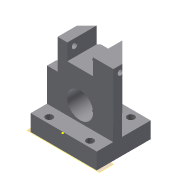
# Autodesk Inventor part: 03_Support_Xslide
Saved by Autodesk Inventor 2019.4 (Build 234330000, 330)
## iProperties
Created: 2021-02-01
Part Number: 03_Support_Xslide
Material: Generic
Document SubType Name: Modeling
Designer: diederichbenedict
Density: 1 g/cm^3
Appearance: Default
Author: diederichbenedict
Autodesk Inventor part; units mm, degrees
ref_plane "YZ Plane" through (0, 0, 0) normal (1, 0, 0) x (0, 1, 0)
ref_plane "XZ Plane" through (0, 0, 0) normal (0, 1, 0) x (-1, 0, 0)
ref_plane "XY Plane" through (0, 0, 0) normal (0, 0, 1) x (1, 0, 0)
ref_plane "Work Plane5" through (16.1538, -3.6432, -7.1) normal (0.0029789, 0.9999956, 0) x (0, 0, 1)
sketch "Sketch5" plane through (16.1538, -3.6432, -7.1) normal (0.0029789, 0.9999956, 0) x (0, 0, 1)
  circle A0 centre (-16.4, -26.2) radius 1.75 projected
  circle A1 centre (-16.4, -6.2) radius 1.75 projected
  line L0 (0, -32.4) -> (6.5, -32.4) projected
  line L1 (6.5, 0) -> (6.5, -32.4) projected
  line L2 (0, 0) -> (6.5, 0) projected
  line L3 (0, 0) -> (0, -32.4) projected
  circle A2 centre (3.6, -6.2) radius 1.75 projected
  circle A3 centre (3.6, -26.2) radius 1.75 projected
  line L4 (-19.9, 0) -> (-19.9, -32.4) projected
  line L5 (6.5, -32.4) -> (-19.9, -32.4)
  line L6 (-19.9, -32.4) -> (-19.9, 0)
  line L7 (-19.9, 0) -> (6.5, 0)
  line L8 (6.5, 0) -> (6.5, -32.4)
  point P0 (7.1, -16.1645)
  constraints: 8 end point, 2 parallel, 1 horizontal, 1 perpendicular
extrude "Extrusion4" add sketch "Sketch5" along normal blind 8
sketch "Sketch7" plane through (16.1776, 4.3568, -7.1) normal (0.0029789, 0.9999956, 0) x (0.9999956, -0.0029789, 0)
  point P0 (-16.1645, -7.1)
sketch "Sketch8" plane through (16.1776, 4.3568, -7.1) normal (0.0029789, 0.9999956, 0) x (0.9999956, -0.0029789, 0)
  circle A0 centre (-26.2, -3.6) radius 1.75 projected
  circle A1 centre (-6.2, -3.6) radius 1.75 projected
  circle A2 centre (-6.2, 16.4) radius 1.75 projected
  circle A3 centre (-26.2, 16.4) radius 1.75 projected
  line L0 (-32.4, -6.5) -> (0, -6.5) projected
  line L1 (0, -6.5) -> (0, 19.9) projected
  line L2 (0, 19.9) -> (-32.4, 19.9) projected
  line L3 (-32.4, 19.9) -> (-32.4, -6.5) projected
  circle A4 centre (-16.2177, 39.3896) radius 1.75 projected
  line L4 (-22.2006, -0.6104) -> (-22.0458, -0.6104) projected
  line L5 (-22.2, -0.6104) -> (-22.2, -0.6104) projected
  line L6 (-22.2, -0.6104) -> (-21.7015, -0.6104) projected
  line L7 (-21.7015, -0.6104) -> (-14.6224, -0.6104) projected
  line L8 (-14.6224, -0.6104) -> (-13.8248, -0.6104) projected
  line L9 (-13.8248, -0.6104) -> (-10.7339, -0.6104) projected
  line L10 (-10.7339, -0.6104) -> (-10.2354, -0.6104) projected
  line L11 (-10.2354, -0.6104) -> (-10.2354, -0.6104) projected
  line L12 (-10.3901, -0.6104) -> (-10.2354, -0.6104) projected
  line L13 (-10.966, -0.6104) -> (-10.3901, -0.6104) projected
  line L14 (-11.1588, -0.6104) -> (-10.966, -0.6104) projected
  line L15 (-11.1588, -0.6104) -> (-11.5034, -0.6104) projected
  line L16 (-11.731, -0.6104) -> (-11.5034, -0.6104) projected
  line L17 (-11.731, -0.6104) -> (-11.731, -0.6104) projected
  line L18 (-11.731, -0.6104) -> (-11.5034, -0.6104) projected
  line L19 (-11.5034, -0.6104) -> (-11.1379, -0.6104) projected
  line L20 (-11.1379, -0.6104) -> (-10.9487, -0.6104) projected
  line L21 (-10.9487, -0.6104) -> (-10.3901, -0.6104) projected
  line L22 (-10.3901, -0.6104) -> (-10.2354, -0.6104) projected
  line L23 (-10.2354, -0.6104) -> (-10.2354, -0.6104) projected
  line L24 (-10.2354, -0.6104) -> (-10.7339, -0.6104) projected
  line L25 (-10.7339, -0.6104) -> (-21.7015, -0.6104) projected
  line L26 (-21.7015, -0.6104) -> (-22.2, -0.6104) projected
  line L27 (-22.2, -0.6104) -> (-22.2, -0.6104) projected
  line L28 (-22.2001, -0.6104) -> (-22.0454, -0.6104) projected
  line L29 (-22.0454, -0.6104) -> (-21.4867, -0.6104) projected
  line L30 (-21.4867, -0.6104) -> (-21.2975, -0.6104) projected
  line L31 (-21.2975, -0.6104) -> (-20.932, -0.6104) projected
  line L32 (-20.932, -0.6104) -> (-20.7045, -0.6104) projected
  line L33 (-20.7045, -0.6104) -> (-20.7045, -0.6104) projected
  line L34 (-20.932, -0.6104) -> (-20.7045, -0.6104) projected
  line L35 (-20.932, -0.6104) -> (-21.2766, -0.6104) projected
  line L36 (-21.4694, -0.6104) -> (-21.2766, -0.6104) projected
  line L37 (-22.0458, -0.6104) -> (-21.4694, -0.6104) projected
  line L38 (-32.4, 19.9) -> (-32.4, -6.5) projected
  line L39 (-32.4, 5.9) -> (-21.4, 16.9)
  line L40 (-21.4, 16.9) -> (-11, 16.9)
  line L41 (-11, 16.9) -> (0, 5.9)
  line L42 (0, -6.5) -> (0, 19.9) projected
  line L43 (0, 1.5) -> (-32.4, 1.5)
  line L44 (-32.4, 5.9) -> (-32.4, -0.0368)
  line L45 (0, 5.9) -> (0, 1.5)
  circle A5 centre (-16.2177, 9.3896) radius 1.75
  circle A6 centre (-16.2177, 9.3896) radius 1.4
  point P0 (-16.1645, -7.1)
  dimension "d25" = 45
  dimension "d26" = 45
  dimension "d27" = 3
  dimension "d28" = 11
  dimension "d29" = 11
  dimension "d30" = 8
  dimension "d46" = 2.8
  constraints: 12 end point, 5 point on line, 3 perpendicular, 2 centre point, 1 coincident, 3 other
  measures "d25" angle of L3 L39
  measures "d26" angle of L1 L41
  measures "d27" distance between parallel lines of L2 L40
  measures "d28" distance from line of L3 L39.end
  measures "d29" distance from line of L1 L40.end
  measures "d30" distance between parallel lines of L0 L43
  measures "d46" diameter of A6
ref_plane "Work Plane7" through (-5.4512, 35.4213, -181.4907) normal (0.0029789, 0.9999956, 0) x (0, 0, 1)
extrude "Extrusion5" add sketch "Sketch8" along normal up to surface (31 mm away) contours L43 L3 L39 L40 L41 L1 | A5
sketch "Sketch9" plane through (16.2699, 35.3566, -8.6) normal (0.0029789, 0.9999956, 0) x (0.9999956, -0.0029789, 0)
  line L0 (-22.2, -2.1104) -> (-22.2, 197.8896) projected
  line L1 (-10.2354, -2.1104) -> (-10.2354, 197.8896) projected
  line L2 (-22.5, 20.2984) -> (-9.9354, 20.2984)
  line L3 (-9.9354, 20.2984) -> (-9.9354, -1.0464)
  line L4 (-9.9354, -1.0464) -> (-22.5, -1.0464)
  line L5 (-22.5, -1.0464) -> (-22.5, 20.2984)
  point P0 (-16.1645, -8.6)
  dimension "d34" = 0.3
  dimension "d35" = 0.3
  constraints: 8 end point, 2 parallel, 1 horizontal, 1 perpendicular
  measures "d34" distance between parallel lines of L0 L5
  measures "d35" distance between parallel lines of L1 L3
ref_plane "Work Plane8" through (-5.4751, 27.4214, -181.4903) normal (-0.0029789, -0.9999956, 0) x (0.9999956, -0.0029789, 0)
extrude "Extrusion6" cut sketch "Sketch9" against normal up to surface (8 mm away)
sketch "Sketch10" plane through (-16.2461, -3.5467, -27) normal (-0.9999956, 0.0029789, 0) x (0, 0, 1)
  line L0 (0, 0) -> (26.4, 0) projected
  line L1 (26.4, 0) -> (26.4, 8) projected
  line L2 (18.4, 8) -> (26.4, 8) projected
  line L3 (0, 0) -> (0, 8) projected
  circle A0 centre (14.8051, 35.8681) radius 1.4
  line L4 (18.4, 8) -> (18.4, 39) projected
  line L5 (18.4, 39) -> (14, 39) projected
  line L6 (14, 8) -> (14, 39) projected
  line L7 (0, 8) -> (14, 8) projected
  point P0 (27, 3.595)
  dimension "d38" = 2.8
  constraints: 1 centre point
  measures "d38" diameter of A0
extrude "Extrusion7" cut sketch "Sketch10" against normal through all contours L6 A0 | A0 L6
sketch "Sketch11" plane through (-16.2223, 4.4533, -8.6) normal (0, 0, 1) x (0.9999956, -0.0029789, 0)
  circle A0 centre (16.2, 7.5) radius 5.65 projected
  circle A1 centre (16.2, 7.5) radius 6.35
  point P0 (16.2355, -4.405)
  dimension "d41" = 0.7
  constraints: 1 centre point
  measures "d41" radial gap between concentric circles of A0 A1
extrude "Extrusion8" cut sketch "Sketch11" against normal through all contours A0 | A1
sketch "Sketch12" plane through (-16.2223, 4.4533, -8.6) normal (0, 0, 1) x (0.9999956, -0.0029789, 0)
  line L0 (3.2, 22.4) -> (-3.8, 22.4) projected
  line L1 (3.2, 22.4) -> (3.2, 72.4) projected
  line L2 (-3.8, 72.4) -> (3.2, 72.4) projected
  line L3 (3.2, 18.4) -> (3.2, 26.4) projected
  line L4 (-2.7347, 16.1972) -> (5.1158, 16.1972)
  line L5 (5.1158, 16.1972) -> (5.1158, 65.2014)
  line L6 (5.1158, 65.2014) -> (-2.7347, 65.2014)
  line L7 (-2.7347, 65.2014) -> (-2.7347, 16.1972)
  line L8 (-3.8, 22.4) -> (-3.8, 72.4) projected
  line L9 (-3.8, 18.4) -> (3.2, 18.4) projected
  line L10 (-3.8, 26.4) -> (-3.8, 18.4) projected
  line L11 (3.2, 26.4) -> (-3.8, 26.4) projected
  point P0 (16.2355, -4.405)
  point P1 (-1.8, 18.4)
  point P2 (-1.8, 26.4)
  constraints: 8 end point, 2 parallel, 1 horizontal, 1 perpendicular
extrude "Extrusion9" cut sketch "Sketch12" against normal through all contours L3 L9 L7 L0 | L0 L7 L11 L1 | L1 L6 L5 L4 L7 L9 L3 | L11 L7 L6 L1
body "Solid2"
